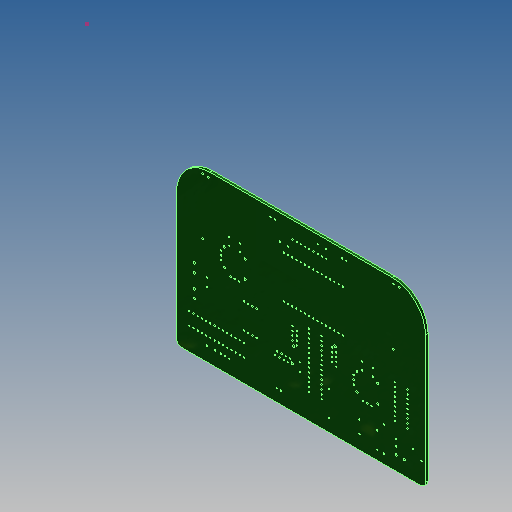
# Autodesk Inventor part: manette_2019.kicad_pcb_Contour
Saved by Autodesk Inventor 2019 (Build 230136000, 136)
## iProperties
Created: 2019-05-20
Part Number: manette_2019.kicad_pcb_Contour
Project: Nom Projet
Material: .
Description: Nom pièce
Document SubType Name: Modeling
Designer: Adel.KAHRIMANOVIC
Authority: brut Ø
Density: 0.001 g/cm^3
Appearance: Contour du circuit imprimé
Author: Adel.KAHRIMANOVIC
Material number: ---
Autodesk Inventor part; units mm, degrees
ref_plane "Plan YZ" through (0, 0, 0) normal (1, 0, 0) x (0, 1, 0)
ref_plane "Plan XZ" through (0, 0, 0) normal (0, 1, 0) x (-1, 0, 0)
ref_plane "Plan XY" through (0, 0, 0) normal (0, 0, 1) x (1, 0, 0)
sketch "Esquisse1" plane through (0, 0, 0) normal (0, 0, 1) x (1, 0, 0)
  point P0 (0, 0)
sketch "Esquisse6" plane through (0, 0, 0) normal (0, 0, 1) x (1, 0, 0)
  arc A0 (55.88, -135.735) -> (58.88, -138.735) centre (58.88, -135.735) ccw
  line L0 (58.88, -138.735) -> (202.88, -138.735)
  arc A1 (202.88, -138.735) -> (205.88, -135.735) centre (202.88, -135.735) ccw
  line L1 (205.88, -135.735) -> (205.88, -58.735)
  arc A2 (205.88, -58.735) -> (185.88, -38.735) centre (185.88, -58.735) ccw
  line L2 (185.88, -38.735) -> (75.88, -38.735)
  arc A3 (75.88, -38.735) -> (55.88, -58.735) centre (75.88, -58.735) ccw
  line L3 (55.88, -58.735) -> (55.88, -135.735)
  circle A4 centre (74.168, -94.615) radius 0.4
  circle A5 centre (74.168, -99.615) radius 0.4
  circle A6 centre (118.11, -53.975) radius 0.4
  circle A7 centre (123.11, -53.975) radius 0.4
  circle A8 centre (130.048, -110.871) radius 0.4
  circle A9 centre (130.048, -115.871) radius 0.4
  circle A10 centre (74.168, -130.175) radius 0.4
  circle A11 centre (79.168, -130.175) radius 0.4
  circle A12 centre (145.97, -43.815) radius 0.4
  circle A13 centre (140.97, -43.815) radius 0.4
  circle A14 centre (176.784, -133.223) radius 0.4
  circle A15 centre (176.784, -123.063) radius 0.4
  circle A16 centre (188.214, -121.92) radius 0.4
  circle A17 centre (198.374, -121.92) radius 0.4
  circle A18 centre (66.548, -90.805) radius 0.65
  circle A19 centre (66.548, -95.885) radius 0.65
  circle A20 centre (66.548, -104.267) radius 0.65
  circle A21 centre (66.548, -109.347) radius 0.65
  circle A22 centre (115.0722, -43.815) radius 0.4
  circle A23 centre (112.5322, -43.815) radius 0.4
  circle A24 centre (158.242, -43.815) radius 0.4
  circle A25 centre (155.702, -43.815) radius 0.4
  circle A26 centre (125.73, -48.895) radius 0.4
  circle A27 centre (128.27, -48.895) radius 0.4
  circle A28 centre (130.81, -48.895) radius 0.4
  circle A29 centre (133.35, -48.895) radius 0.4
  circle A30 centre (135.89, -48.895) radius 0.4
  circle A31 centre (138.43, -48.895) radius 0.4
  circle A32 centre (140.97, -48.895) radius 0.4
  circle A33 centre (143.51, -48.895) radius 0.4
  circle A34 centre (146.05, -48.895) radius 0.4
  circle A35 centre (193.294, -130.175) radius 0.65
  circle A36 centre (188.214, -130.175) radius 0.65
  circle A37 centre (116.205, -131.445) radius 0.4
  circle A38 centre (118.745, -131.445) radius 0.4
  circle A39 centre (152.146, -102.235) radius 0.4
  circle A40 centre (149.606, -100.965) radius 0.4
  circle A41 centre (152.146, -99.695) radius 0.4
  circle A42 centre (149.606, -98.425) radius 0.4
  circle A43 centre (152.146, -97.155) radius 0.4
  circle A44 centre (149.606, -95.885) radius 0.4
  circle A45 centre (152.146, -94.615) radius 0.4
  circle A46 centre (149.606, -93.345) radius 0.4
  circle A47 centre (125.73, -94.107) radius 0.4
  circle A48 centre (128.27, -95.377) radius 0.4
  circle A49 centre (125.73, -96.647) radius 0.4
  circle A50 centre (128.27, -97.917) radius 0.4
  circle A51 centre (125.73, -99.187) radius 0.4
  circle A52 centre (128.27, -100.457) radius 0.4
  circle A53 centre (125.73, -101.727) radius 0.4
  circle A54 centre (128.27, -102.997) radius 0.4
  circle A55 centre (124.206, -111.887) radius 0.4
  circle A56 centre (122.936, -114.427) radius 0.4
  circle A57 centre (121.666, -111.887) radius 0.4
  circle A58 centre (120.396, -114.427) radius 0.4
  circle A59 centre (119.126, -111.887) radius 0.4
  circle A60 centre (117.856, -114.427) radius 0.4
  circle A61 centre (116.586, -111.887) radius 0.4
  circle A62 centre (115.316, -114.427) radius 0.4
  circle A63 centre (82.63, -76.235) radius 0.45
  circle A64 centre (82.63, -78.735) radius 0.45
  circle A65 centre (82.63, -81.235) radius 0.45
  circle A66 centre (90.88, -86.985) radius 0.45
  circle A67 centre (88.38, -86.985) radius 0.45
  circle A68 centre (93.38, -86.985) radius 0.45
  circle A69 centre (87.63, -71.285) radius 0.4
  circle A70 centre (94.13, -71.285) radius 0.4
  circle A71 centre (94.13, -66.785) radius 0.4
  circle A72 centre (87.63, -66.785) radius 0.4
  circle A73 centre (167.63, -91.785) radius 0.4
  circle A74 centre (174.13, -91.785) radius 0.4
  circle A75 centre (174.13, -96.285) radius 0.4
  circle A76 centre (167.63, -96.285) radius 0.4
  circle A77 centre (173.38, -111.985) radius 0.45
  circle A78 centre (168.38, -111.985) radius 0.45
  circle A79 centre (170.88, -111.985) radius 0.45
  circle A80 centre (162.63, -106.235) radius 0.45
  circle A81 centre (162.63, -103.735) radius 0.45
  circle A82 centre (162.63, -101.235) radius 0.45
  circle A83 centre (166.116, -130.429) radius 0.4
  circle A84 centre (166.116, -122.809) radius 0.4
  circle A85 centre (188.214, -125.73) radius 0.4
  circle A86 centre (203.454, -125.73) radius 0.4
  circle A87 centre (180.848, -117.983) radius 0.4
  circle A88 centre (180.848, -133.223) radius 0.4
  circle A89 centre (147.828, -115.951) radius 0.4
  circle A90 centre (147.828, -131.191) radius 0.4
  circle A91 centre (71.63, -41.735) radius 0.5
  circle A92 centre (75.13, -41.735) radius 0.5
  circle A93 centre (71.63, -75.735) radius 0.5
  circle A94 centre (186.63, -41.735) radius 0.5
  circle A95 centre (190.13, -41.735) radius 0.5
  circle A96 centre (186.63, -75.735) radius 0.5
  circle A97 centre (156.085, -58.37) radius 0.4
  circle A98 centre (153.545, -58.37) radius 0.4
  circle A99 centre (151.005, -58.37) radius 0.4
  circle A100 centre (148.465, -58.37) radius 0.4
  circle A101 centre (145.925, -58.37) radius 0.4
  circle A102 centre (143.385, -58.37) radius 0.4
  circle A103 centre (140.845, -58.37) radius 0.4
  circle A104 centre (138.305, -58.37) radius 0.4
  circle A105 centre (135.765, -58.37) radius 0.4
  circle A106 centre (133.225, -58.37) radius 0.4
  circle A107 centre (130.685, -58.37) radius 0.4
  circle A108 centre (128.145, -58.37) radius 0.4
  circle A109 centre (125.605, -58.37) radius 0.4
  circle A110 centre (123.065, -58.37) radius 0.4
  circle A111 centre (120.525, -58.37) radius 0.4
  circle A112 centre (156.085, -83.87) radius 0.4
  circle A113 centre (128.145, -83.87) radius 0.4
  circle A114 centre (143.385, -83.87) radius 0.4
  circle A115 centre (133.225, -83.87) radius 0.4
  circle A116 centre (153.545, -83.87) radius 0.4
  circle A117 centre (148.465, -83.87) radius 0.4
  circle A118 centre (140.845, -83.87) radius 0.4
  circle A119 centre (130.685, -83.87) radius 0.4
  circle A120 centre (125.605, -83.87) radius 0.4
  circle A121 centre (145.925, -83.87) radius 0.4
  circle A122 centre (138.305, -83.87) radius 0.4
  circle A123 centre (123.065, -83.87) radius 0.4
  circle A124 centre (151.005, -83.87) radius 0.4
  circle A125 centre (120.525, -83.87) radius 0.4
  circle A126 centre (135.765, -83.87) radius 0.4
  circle A127 centre (63.5, -125.095) radius 0.4
  circle A128 centre (96.52, -117.475) radius 0.4
  circle A129 centre (66.04, -125.095) radius 0.4
  circle A130 centre (93.98, -117.475) radius 0.4
  circle A131 centre (68.58, -125.095) radius 0.4
  circle A132 centre (91.44, -117.475) radius 0.4
  circle A133 centre (71.12, -125.095) radius 0.4
  circle A134 centre (88.9, -117.475) radius 0.4
  circle A135 centre (73.66, -125.095) radius 0.4
  circle A136 centre (86.36, -117.475) radius 0.4
  circle A137 centre (76.2, -125.095) radius 0.4
  circle A138 centre (83.82, -117.475) radius 0.4
  circle A139 centre (78.74, -125.095) radius 0.4
  circle A140 centre (81.28, -117.475) radius 0.4
  circle A141 centre (81.28, -125.095) radius 0.4
  circle A142 centre (78.74, -117.475) radius 0.4
  circle A143 centre (83.82, -125.095) radius 0.4
  circle A144 centre (76.2, -117.475) radius 0.4
  circle A145 centre (86.36, -125.095) radius 0.4
  circle A146 centre (73.66, -117.475) radius 0.4
  circle A147 centre (88.9, -125.095) radius 0.4
  circle A148 centre (71.12, -117.475) radius 0.4
  circle A149 centre (91.44, -125.095) radius 0.4
  circle A150 centre (68.58, -117.475) radius 0.4
  circle A151 centre (93.98, -125.095) radius 0.4
  circle A152 centre (66.04, -117.475) radius 0.4
  circle A153 centre (96.52, -125.095) radius 0.4
  circle A154 centre (63.5, -117.475) radius 0.4
  circle A155 centre (135.636, -90.551) radius 0.4
  circle A156 centre (143.256, -123.571) radius 0.4
  circle A157 centre (135.636, -93.091) radius 0.4
  circle A158 centre (143.256, -121.031) radius 0.4
  circle A159 centre (135.636, -95.631) radius 0.4
  circle A160 centre (143.256, -118.491) radius 0.4
  circle A161 centre (135.636, -98.171) radius 0.4
  circle A162 centre (143.256, -115.951) radius 0.4
  circle A163 centre (135.636, -100.711) radius 0.4
  circle A164 centre (143.256, -113.411) radius 0.4
  circle A165 centre (135.636, -103.251) radius 0.4
  circle A166 centre (143.256, -110.871) radius 0.4
  circle A167 centre (135.636, -105.791) radius 0.4
  circle A168 centre (143.256, -108.331) radius 0.4
  circle A169 centre (135.636, -108.331) radius 0.4
  circle A170 centre (143.256, -105.791) radius 0.4
  circle A171 centre (135.636, -110.871) radius 0.4
  circle A172 centre (143.256, -103.251) radius 0.4
  circle A173 centre (135.636, -113.411) radius 0.4
  circle A174 centre (143.256, -100.711) radius 0.4
  circle A175 centre (135.636, -115.951) radius 0.4
  circle A176 centre (143.256, -98.171) radius 0.4
  circle A177 centre (135.636, -118.491) radius 0.4
  circle A178 centre (143.256, -95.631) radius 0.4
  circle A179 centre (135.636, -121.031) radius 0.4
  circle A180 centre (143.256, -93.091) radius 0.4
  circle A181 centre (135.636, -123.571) radius 0.4
  circle A182 centre (143.256, -90.551) radius 0.4
  circle A183 centre (187.452, -92.583) radius 0.4
  circle A184 centre (195.072, -112.903) radius 0.4
  circle A185 centre (187.452, -95.123) radius 0.4
  circle A186 centre (195.072, -110.363) radius 0.4
  circle A187 centre (187.452, -97.663) radius 0.4
  circle A188 centre (195.072, -107.823) radius 0.4
  circle A189 centre (187.452, -100.203) radius 0.4
  circle A190 centre (195.072, -105.283) radius 0.4
  circle A191 centre (187.452, -102.743) radius 0.4
  circle A192 centre (195.072, -102.743) radius 0.4
  circle A193 centre (187.452, -105.283) radius 0.4
  circle A194 centre (195.072, -100.203) radius 0.4
  circle A195 centre (187.452, -107.823) radius 0.4
  circle A196 centre (195.072, -97.663) radius 0.4
  circle A197 centre (187.452, -110.363) radius 0.4
  circle A198 centre (195.072, -95.123) radius 0.4
  circle A199 centre (187.452, -112.903) radius 0.4
  circle A200 centre (195.072, -92.583) radius 0.4
  circle A201 centre (104.14, -111.125) radius 0.45
  circle A202 centre (101.6, -111.125) radius 0.45
  circle A203 centre (99.06, -111.125) radius 0.45
  circle A204 centre (96.52, -111.125) radius 0.45
  circle A205 centre (96.52, -95.885) radius 0.45
  circle A206 centre (99.06, -95.885) radius 0.45
  circle A207 centre (101.6, -95.885) radius 0.45
  circle A208 centre (104.14, -95.885) radius 0.45
  circle A209 centre (82.59, -130.175) radius 0.4
  circle A210 centre (85.09, -130.175) radius 0.4
  circle A211 centre (87.59, -130.175) radius 0.4
  circle A212 centre (151.406, -91.945) radius 0.75
  circle A213 centre (126.47, -104.397) radius 0.75
  circle A214 centre (125.606, -113.687) radius 0.75
  circle A215 centre (84.63, -73.435) radius 0.65
  circle A216 centre (84.63, -84.035) radius 0.65
  circle A217 centre (97.13, -84.035) radius 0.65
  circle A218 centre (97.13, -73.435) radius 0.65
  circle A219 centre (177.13, -98.435) radius 0.65
  circle A220 centre (177.13, -109.035) radius 0.65
  circle A221 centre (164.63, -109.035) radius 0.65
  circle A222 centre (164.63, -98.435) radius 0.65
  constraints: 223 centre point, 8 end point, 8 point on circle
extrude "manette_2019.kicad_pcb_Contour" add sketch "Esquisse6" along normal blind 1.6
